Autodesk Fusion 360 part; units mm, degrees
(part 4 of 4)
sketch "Sketch3" plane through (0, 0, 0) normal (1, 0, 0) x (0, 0, -1)
  line L0 (150, -50) -> (150, 100)
  line L1 (150, 100) -> (0, 100)
  line L2 (0, 100) -> (0, -50)
  line L3 (0, -50) -> (150, -50)
  line L4 (65, 80) -> (65, -20)
  line L5 (85, 80) -> (85, -20)
  arc A0 (85, 80) -> (65, 80) centre (75, 80) ccw
  arc A1 (65, -20) -> (85, -20) centre (75, -20) ccw
  dimension "d5" = 100
  dimension "d6" = 100
  dimension "d9" = 20
  dimension "d10" = 65
  constraint vertical L4
  constraint vertical L5
  constraint tangent L5 A0
  constraint tangent L4 A0
  constraint tangent L5 A1
  measures "d5" distance of L4.start L4.end
  measures "d6" distance of L5.start L5.end
  measures "d9" distance of L4.start L5.start
  measures "d10" horizontal distance of origin L4.start
extrude "Extrude2" cut sketch "Sketch3" against normal blind 60 contours L4 L5 A0 A1 bodies 1
sketch "草图4" plane through (-7, 0, 0) normal (-1, 0, 0) x (0, 0, 1)
  line L0 (-65, 80) -> (-65, -20)
  arc A0 (-85, -20) -> (-65, -20) centre (-75, -20) ccw
  line L1 (-85, -20) -> (-85, 80)
  arc A1 (-65, 80) -> (-85, 80) centre (-75, 80) ccw
  line L2 (0, -50) -> (0, 100)
  line L3 (0, 100) -> (-150, 100)
  line L4 (-150, 100) -> (-150, -50)
  line L5 (-150, -50) -> (0, -50)
  circle A2 centre (-75, 95) radius 2.5
  dimension "d13" = 5
  dimension "d14" = 5
  measures "d13" diameter of A2
  measures "d14" distance of L3 A2.centre
extrude "拉伸3" cut sketch "草图4" against normal through all contours A2 bodies 1
sketch "草图5" plane through (0, 0, 0) normal (1, 0, 0) x (0, 0, -1)
  circle A0 centre (75, 95) radius 2.5
  line L0 (65, -20) -> (65, 80)
  arc A1 (85, 80) -> (65, 80) centre (75, 80) ccw
  line L1 (85, 80) -> (85, -20)
  arc A2 (65, -20) -> (85, -20) centre (75, -20) ccw
  line L2 (150, -50) -> (150, 100)
  line L3 (150, 100) -> (0, 100)
  line L4 (0, 100) -> (0, -50)
  line L5 (0, -50) -> (150, -50)
  line L6 (65, 80) -> (67.8191, 78.9739)
  line L7 (65, 80) -> (70, 80) construction
  line L8 (67.8191, 78.9739) -> (67.8191, 77.9739)
  line L9 (67.8191, 77.9739) -> (65, 76.9479)
  line L10 (67.8191, 77.9739) -> (74.6985, 77.9739) construction
  line L11 (65, 80) -> (65, 76.9479)
  dimension "d16" = 20
  dimension "d17" = 3
  dimension "d18" = 1
  dimension "d19" = 160
  dimension "d20" = 3
  constraint horizontal L7
  constraint coincident L0.end A1.end
  constraint vertical L8
  constraint horizontal L10
  measures "d16" angle of L6 L7
  measures "d17" distance of L0.end L6.end
  measures "d18" distance of L6.end L8.end
  measures "d19" angle of L9 L10
  measures "d20" distance of L8.end L9.end
extrude "拉伸4" add sketch "草图5" against normal blind 7 separate body contours L0 L6 L8 L9 L11 makes body 2
pattern_linear "R-阵列1" count 16 spacing 6.3333 along (0, -1, 0) of "拉伸4" makes body 3 at (-2.3333, 71.6319, -65) makes body 4 at (-4.6667, 65.2986, -65) makes body 5 at (-2.3333, 58.9653, -65) makes body 6 at (-2.3333, 52.6319, -65) makes body 7 at (-2.3333, 46.2986, -65) makes body 8 at (-2.3333, 39.9653, -65) makes body 9 at (-2.3333, 33.6319, -65) makes body 10 at (-4.6667, 27.2986, -65) makes body 11 at (-2.3333, 20.9653, -65) makes body 12 at (-2.3333, 14.6319, -65) makes body 13 at (-2.3333, 8.2986, -65) makes body 14 at (-2.3333, 1.9653, -65) makes body 15 at (-2.3333, -4.3681, -65) makes body 16 at (-2.3333, -10.7014, -65) makes body 17 at (-2.3333, -17.0347, -65)
thread "螺纹1" "ISO Metric profile 5.0 M5x0.8 6H" major diameter 5.12 minor diameter 4.234 pitch 0.8 angle 60 resizes the face on face at (-2.3333, 94.0289, -77.3037) on bodies 1
